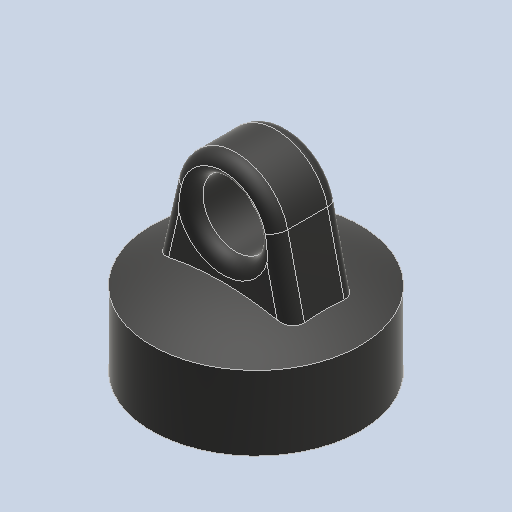
# Autodesk Inventor part: タミヤダンパー1
Saved by Autodesk Inventor 2023 (Build 270158030, 158C)
## iProperties
Part Number: タミヤダンパー1
Material: アセタール樹脂、黒
Document SubType Name: Modeling
Designer: 雪村
Density: 1.425 g/cm^3
Appearance: 滑らか - 黒
Mass: 1.52347 g
Surface Area: 10.0595 cm^2
Volume: 1.0691 cm^3
Author: 雪村
Autodesk Inventor part; units mm, degrees
ref_plane "YZ Plane" through (0, 0, 0) normal (1, 0, 0) x (0, 1, 0)
ref_plane "XZ Plane" through (0, 0, 0) normal (0, 1, 0) x (-1, 0, 0)
ref_plane "XY Plane" through (0, 0, 0) normal (0, 0, 1) x (1, 0, 0)
sketch "スケッチ1" plane through (0, 0, 0) normal (0, 0, 1) x (1, 0, 0)
  circle A0 centre (0, 0) radius 7.875
  dimension "d0" = 15.75
  constraints: 1 centre point, 1 coincident
  measures "d0" diameter of A0
extrude "押し出し1" add sketch "スケッチ1" along normal blind 5.6
sketch "スケッチ2" plane through (0, 0, 0) normal (0, 1, 0) x (-1, 0, 0)
  line L0 (7.875, 5.6) -> (-7.875, 5.6)
  circle A0 centre (0, 11.033601) radius 2.5
  arc A1 (3.89748, 11.933405) -> (-3.89748, 11.933405) centre (0, 11.033601) ccw
  line L1 (3.89748, 11.933405) -> (5.359662, 5.6)
  line L2 (-3.89748, 11.933405) -> (-5.359662, 5.6)
  line L3 (0, 11.033601) -> (0.809241, 11.033601)
  point P0 (0, 0)
  dimension "d3" = 5
  dimension "d4" = 1.5
  dimension "d5" = 103
  dimension "d6" = 103
  dimension "d7" = 6.5
  constraints: 6 end point, 2 centre point, 2 point on circle, 2 point on line, 2 tangent, 1 horizontal, 1 vertical alignment
  measures "d3" diameter of A0
  measures "d4" radial gap between concentric circles of A0 A1
  measures "d5" angle of L3 L1
  measures "d6" angle of L2 L3
  measures "d7" distance of L1.start L1.end
extrude "押し出し2" add sketch "スケッチ2" along normal mid plane 5
sketch "スケッチ3" plane through (0, 0, 0) normal (0, 1, 0) x (-1, 0, 0)
  line L0 (7.875, 5.6) -> (-7.875, 5.6)
  line L1 (0, 5.6) -> (0, 7.215649)
  arc A0 (7.875, 5.6) -> (0, 7.215649) centre (0, -12.784351) ccw
  point P0 (0, 0)
  dimension "d10" = 20
  constraints: 3 end point, 2 point on circle, 1 centre point, 1 midpoint, 1 vertical, 1 other
  measures "d10" radius of A0
revolve "回転1" add sketch "スケッチ3" angle 360 about axis through (0, 0, 5.6) along (0, 0, 1)
sketch "スケッチ4" plane through (0, 0, 0) normal (0, 0, -1) x (-1, 0, 0)
  circle A0 centre (0, 0) radius 5.5
  dimension "d12" = 11
  constraints: 1 centre point, 1 coincident
  measures "d12" diameter of A0
extrude "押し出し3" cut sketch "スケッチ4" against normal blind 4
fillet "フィレット1" radius 1 8 edges at (0, -2.5, 15.0336) (4.5397, -2.5, 9.1518) (-4.5397, -2.5, 9.1518) (2.5, -2.5, 11.0336) (0, 2.5, 15.0336) (-4.5397, 2.5, 9.1518) (4.5397, 2.5, 9.1518) (2.5, 2.5, 11.0336)
equation "\"d6\" = d5"
